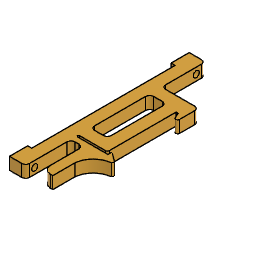
Parametric DIN Rail Mount (Autodesk Fusion 360 design; units mm, degrees)
Autodesk Fusion 360 part; units mm, degrees
note: some values were not read from the file. Set by a fixed rule: which sketch regions a step uses.
sketch "Sketch1" plane through (0, 0, 0) normal (0, 0, 1) x (1, 0, 0)
  line L0 (0, 0) -> (0, 40)
  line L1 (0, 40) -> (0, 41.5)
  line L2 (0, 41.5) -> (0, 44.5)
  line L3 (0, 44.5) -> (-6, 44.5)
  line L4 (-6, 44.5) -> (-6, 0)
  line L5 (-6, 0) -> (0, 0)
  line L6 (0, 0) -> (0, 22.871)
  line L7 (0, 22.871) -> (18.28, 22.871)
  line L8 (18.28, 22.871) -> (18.28, 9.411)
  line L9 (0, 0) -> (14.28, 0)
  line L10 (14.28, 0) -> (14.28, 22.871)
  line L11 (14.28, 22.871) -> (14.28, 15.696)
  line L12 (14.28, 15.696) -> (15.28, 15.696)
  line L13 (15.28, 15.696) -> (18.28, 9.411)
  line L14 (-6, -44.5) -> (-6, 0)
  line L15 (0, 0) -> (0, -40)
  line L16 (0, -44.5) -> (-6, -44.5)
  line L17 (0, -41.5) -> (0, -44.5)
  line L18 (0, -40) -> (0, -41.5)
  line L19 (14.28, 15.696) -> (14.28, -19.304)
  line L20 (14.28, -19.304) -> (14.28, -18.304)
  line L21 (14.28, -18.304) -> (0, -18.304)
  line L22 (0, -18.304) -> (0, -19.304)
  line L23 (0, -19.304) -> (15.55, -19.304)
  line L24 (15.55, -19.304) -> (15.55, -17.304)
  line L25 (0, -19.304) -> (0, -22.065)
  line L26 (0, -22.065) -> (22.064, -22.065)
  line L27 (22.064, -22.065) -> (15.55, -17.304)
  line L28 (-6, 44.5) -> (-6, 41.5)
  line L29 (-6, 41.5) -> (-6, 40)
  line L30 (-6, 40) -> (-6, 35.5)
  line L31 (-6, 35.5) -> (0, 35.5)
  line L32 (-6, 35.5) -> (-8, 35.5)
  line L33 (-6, 44.5) -> (-8, 44.5)
  line L34 (-8, 44.5) -> (-8, 35.5)
  line L35 (-8, -44.5) -> (-8, -35.5)
  line L36 (-6, -44.5) -> (-8, -44.5)
  line L37 (-6, -35.5) -> (-8, -35.5)
  line L38 (22.064, -22.065) -> (17.064, -22.065)
  line L39 (0, -22.065) -> (6, -22.065)
  line L40 (6, -22.065) -> (6, -42.065)
  line L41 (6, -42.065) -> (11, -42.065)
  line L42 (11, -42.065) -> (11, -22.065)
  arc A0 (22.064, -22.065) -> (11, -31.0949) centre (21.005, -32.0606) ccw
  arc A1 (22.6081, -16.9297) -> (5.8598, -30.5987) centre (21.005, -32.0606) ccw
  dimension "d2" = 40
  dimension "d6" = 1.5
  dimension "d7" = 3
  dimension "d8" = 6
  dimension "d10" = 22.871
  dimension "d12" = 18.28
  dimension "d13" = 13.46
  dimension "d14" = 14.28
  dimension "d15" = 7.175
  dimension "d16" = 1
  dimension "d18" = 35
  dimension "d19" = 1
  dimension "d20" = 1
  dimension "d21" = 15.55
  dimension "d22" = 2
  dimension "d23" = 2.761
  dimension "d24" = 22.064
  dimension "d32" = 3
  dimension "d33" = 1.5
  dimension "d34" = 4.5
  dimension "d35" = 2
  dimension "d36" = 2
  dimension "d98" = 6
  dimension "d99" = 20
  dimension "d100" = 5
  dimension "d105" = 5.1641
  constraint coincident L0.start L5.end
  constraint vertical L0
  constraint parallel L0 L1
  constraint parallel L1 L2
  constraint perpendicular L2 L3
  constraint perpendicular L3 L4
  constraint perpendicular L0 L5
  constraint coincident L0 L6.end
  constraint perpendicular L6 L7
  constraint perpendicular L7 L8
  constraint horizontal L9
  constraint coincident L7 L10.end
  constraint perpendicular L7 L10
  constraint perpendicular L7 L11
  constraint perpendicular L10 L12
  constraint symmetric L0.start L5 L6.start
  constraint symmetric L0.end L5 L15.end
  constraint symmetric L1.end L5 L17.start
  constraint symmetric L2.end L5 L16.start
  constraint symmetric L3.end L5 L14.start
  constraint symmetric L4.end L5 L14.end
  constraint perpendicular L9 L19
  constraint parallel L19 L20
  constraint coincident L15 L21.end
  constraint perpendicular L15 L21
  constraint perpendicular L21 L22
  constraint perpendicular L15 L23
  constraint perpendicular L23 L24
  constraint perpendicular L23 L25
  constraint perpendicular L15 L26
  constraint perpendicular L3 L28
  constraint parallel L4 L29
  constraint coincident L4 L30.end
  constraint coincident L0 L31.end
  constraint perpendicular L0 L31
  constraint perpendicular L4 L32
  constraint perpendicular L30 L33
  constraint symmetric L5 L30.end L37.start
  constraint symmetric L5 L32.end L35.end
  constraint symmetric L5 L33.end L35.start
  constraint perpendicular L39 L40
  constraint perpendicular L40 L41
  constraint vertical L42
  constraint coincident L42 A0.end
  measures "d2" distance of L0.start L0.end
  measures "d6" distance of L0.end L1.end
  measures "d7" distance of L1.end L2.end
  measures "d8" distance of L2.end L3.end
  measures "d10" distance of L0.start L6.end
  measures "d12" distance of L6.end L7.end
  measures "d13" distance of L7.end L8.end
  measures "d14" distance of L0.start L9.end
  measures "d15" distance of L10.end L11.end
  measures "d16" distance of L11.end L12.end
  measures "d18" distance of L11.end L19.end
  measures "d19" distance of L19.end L20.end
  measures "d20" distance of L21.end L22.end
  measures "d21" distance of L22.end L23.end
  measures "d22" distance of L23.end L24.end
  measures "d23" distance of L22.end L25.end
  measures "d24" distance of L25.end L26.end
  measures "d32" distance of L3.end L28.end
  measures "d33" distance of L28.end L29.end
  measures "d34" distance of L29.end L30.end
  measures "d35" distance of L30.end L32.end
  measures "d36" distance of L3.end L33.end
  measures "d98" distance of L25.end L39.end
  measures "d99" distance of L39.end L40.end
  measures "d100" distance of L40.end L41.end
extrude "Extrude1" add sketch "Sketch1" along normal blind 6 contours L0 L4 L5 L6 L31 | L5 L14 L15 L16 L17 L18 L22 L25 | L0 L6 L7 L9 L10 L11 L19 | L9 L15 L19 L21 | L0 L1 L2 L3 L4 L28 L29 L30 L31 | L7 L8 L10 L11 L12 L13 | L4 L28 L29 L30 L32 L33 L34 | L14 L35 L36 L37 | L15 L23 L25 L26 L39 A1 | L23 L24 L26 L27 L38 A0 A1 | L24 L27 A1 | L26 L40 A1 | L26 L40 L41 L42 A1 | L26 L38 L42 A0 | L26 L38 A0
sketch "Sketch4" plane through (-8, 0, 0) normal (-1, 0, 0) x (0, -1, 0)
  line L0 (-44.5, 0) -> (-35.5, 0)
  line L1 (-35.5, 0) -> (-35.5, 6)
  line L2 (-35.5, 6) -> (-44.5, 6)
  line L3 (-44.5, 6) -> (-44.5, 0)
  line L4 (-44.5, 0) -> (-35.5, 6)
  line L5 (35.5, 0) -> (44.5, 6)
  circle A0 centre (-40, 3) radius 1.5
  circle A1 centre (40, 3) radius 1.5
  point P0 (35.5, 0)
  point P1 (44.5, 6)
  dimension "d53" = 3
  dimension "d54" = 3
  constraint coincident L0.start L3.end
  constraint coincident L1.end L2.start
  constraint coincident P0 L5.start
  constraint coincident P1 L5.end
  constraint midpoint L4 A0.centre
  constraint midpoint L5 A1.centre
  measures "d53" diameter of A0
  measures "d54" diameter of A1
extrude "Extrude4" cut sketch "Sketch4" against normal up to surface (8 mm away) contours L4 A0 | L4 A0 | L5 A1 | L5 A1
sketch "Sketch6" plane through (0, 0, 6) normal (0, 0, 1) x (-1, 0, 0)
  line L0 (0, 44.5) -> (0, 22.065)
  line L1 (0, 22.065) -> (-6, 22.065)
  line L2 (-22.064, 22.065) -> (-15.55, 17.304)
  line L3 (-15.55, 17.304) -> (-15.55, 19.304)
  line L4 (-15.55, 19.304) -> (0, 19.304)
  line L5 (0, 19.304) -> (0, 18.304)
  line L6 (0, 18.304) -> (-14.28, 18.304)
  line L7 (-14.28, 18.304) -> (-14.28, -15.696)
  line L8 (-14.28, -15.696) -> (-15.28, -15.696)
  line L9 (-15.28, -15.696) -> (-18.28, -9.411)
  line L10 (-18.28, -9.411) -> (-18.28, -22.871)
  line L11 (-18.28, -22.871) -> (0, -22.871)
  line L12 (0, -22.871) -> (0, -44.5)
  line L13 (0, -44.5) -> (8, -44.5)
  line L14 (8, -44.5) -> (8, -35.5)
  line L15 (8, -35.5) -> (6, -35.5)
  line L16 (6, -35.5) -> (6, 35.5)
  line L17 (6, 35.5) -> (8, 35.5)
  line L18 (8, 35.5) -> (8, 44.5)
  line L19 (8, 44.5) -> (0, 44.5)
  line L20 (-14.28, 18.304) -> (6, 18.304)
  line L21 (-14.28, -15.696) -> (-14.28, -22.871)
  line L22 (-14.28, -22.871) -> (6, -22.871)
  line L23 (6, -22.871) -> (6, 18.304)
  line L24 (6, 18.304) -> (-14.28, 18.304)
  line L25 (-14.28, 18.304) -> (-14.28, -22.871)
  line L26 (-8.28, -16.871) -> (0, -16.871)
  line L27 (0, -16.871) -> (0, 12.304)
  line L28 (0, 12.304) -> (-8.28, 12.304)
  line L29 (-8.28, 12.304) -> (-8.28, -16.871)
  line L30 (-6, 22.065) -> (-6, 42.065)
  line L31 (-6, 42.065) -> (-11, 42.065)
  line L32 (-11, 42.065) -> (-11, 31.0949)
  arc A0 (-19.946, 22.065) -> (-11, 31.0949) centre (-21.005, 32.0606) ccw
  line L33 (-19.946, 22.065) -> (-22.064, 22.065)
  dimension "d62" = -6
  constraint coincident L6.end L7.start
  constraint coincident L16 L20.end
  constraint perpendicular L16 L20
  constraint coincident L7.end L8.start
  constraint coincident L11 L21.end
  constraint perpendicular L11 L21
  constraint horizontal L22
  constraint vertical L23
  constraint horizontal L24
  constraint vertical L25
extrude "Extrude6" cut sketch "Sketch6" against normal up to surface (6 mm away) contours L26 L27 L28 L29
fillet "Fillet7" radius 2 10 edges at (0, 44.5, 3) (0, -44.5, 3) (0, 16.871, 3) (0, -12.304, 3) (8.28, -12.304, 3) (8.28, 16.871, 3) (0, -22.065, 3) (6, -22.065, 3) (0, 22.871, 3) (18.28, 22.871, 3)
fillet "Fillet9" radius 0.9 2 edges at (22.064, -22.065, 3) (18.28, 9.411, 3)
fillet "Fillet11" radius 1 1 edges at (14.28, -18.304, 3)
fillet "Fillet12" radius 0.3 1 edges at (15.55, -17.304, 3)
fillet "Fillet13" radius 0.5 2 edges at (0, -18.304, 3) (0, -19.304, 3)
fillet "Fillet19" radius 4 1 edges at (6, -42.065, 3)
equation "Calculated_Distance_Between_Holes = min(200 mm; max(50 mm; Distance_Between_Holes))" comment "DO NOT EDIT"
equation "d2 = Calculated_Distance_Between_Holes / 2"
equation "Thickness = 6 mm"
equation "Screw_Hole_Diameter = 3 mm"
equation "d6 = Screw_Hole_Diameter / 2"
equation "d8 = Thickness"
equation "Calculated_Height = min(200 mm; max(6 mm; Width))" comment "DO NOT EDIT"
equation "d26 = Calculated_Height"
equation "Calculated_Pad_Height = min(200 mm; max(0.001 mm; Pad_Height))" comment "DO NOT SET TO 0, if no height is needed set to 0.001 mm"
equation "d33 = Screw_Hole_Diameter / 2"
equation "d34 = 3 mm + Screw_Hole_Diameter / 2"
equation "d35 = Calculated_Pad_Height"
equation "d36 = Calculated_Pad_Height"
equation "d53 = Screw_Hole_Diameter"
equation "d54 = Screw_Hole_Diameter"
equation "Distance_Between_Holes = 80 mm"
equation "Width = 6 mm"
equation "Pad_Height = 2 mm"
